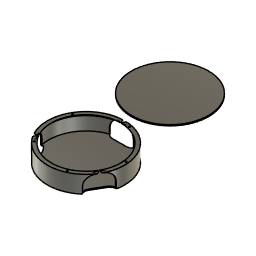
Robotica Volledige Robot3 v2 (Autodesk Fusion 360 design; units mm, degrees)
Autodesk Fusion 360 part; units mm, degrees
sketch "Sketch1" plane through (0, 0, 0) normal (0, 0, 1) x (1, 0, 0)
  circle A0 centre (0, 0) radius 110 construction
  circle A1 centre (0, 0) radius 105.5
  line L0 (-15, 90.5) -> (15, 90.5)
  line L1 (15, 90.5) -> (15, 27.5)
  line L2 (15, 27.5) -> (-15, 27.5)
  line L3 (-15, 27.5) -> (-15, 90.5)
  circle A2 centre (0, 0) radius 102.5
  spline S0 degree 5 poles (-32.987289, 97.046838) (-32.40075, 96.649596) (-31.292492, 95.840182) (-29.823347, 94.581605) (-27.997387, 92.904069) (-24.704967, 91.250774) (-19.527486, 90.398038) (-12.348654, 90.46258) (-5.577784, 90.79374) (-0.094558, 91.003458) (4.346465, 90.964526) (8.472499, 90.723353) (13.019743, 90.460618) (18.177004, 90.44585) (23.049454, 90.978092) (27.290126, 92.192845) (30.008132, 93.760088) (31.651296, 95.273016) (32.571175, 96.430723) (32.987289, 97.046838) knots 0 0 0 0 0 0 0.06666667 0.13333333 0.2 0.26666667 0.33333333 0.4 0.46666667 0.53333333 0.6 0.66666667 0.73333333 0.8 0.86666667 0.93333333 1 1 1 1 1 1
  line L4 (8, 90.5) -> (22, 90.5)
  line L5 (-37.716487, 100.249751) -> (-28.258092, 93.843924)
  line L6 (-24.570837, 90.5) -> (-5.429163, 90.5)
  line L7 (-70.875299, -58.240381) -> (-85.875299, -32.259619)
  line L8 (-16.315699, -26.740381) -> (-70.875299, -58.240381)
  line L9 (-85.875299, -32.259619) -> (-31.315699, -0.759619)
  line L10 (-31.315699, -0.759619) -> (-16.315699, -26.740381)
  spline S1 degree 5 poles (-67.551382, -77.091249) (-67.500631, -76.384671) (-67.353787, -75.020184) (-66.998399, -73.118579) (-66.45859, -70.698483) (-66.673005, -67.020516) (-68.523255, -62.110318) (-72.168565, -55.925538) (-75.840794, -50.227373) (-78.764027, -45.583618) (-80.950823, -41.718114) (-82.804978, -38.024277) (-84.851065, -33.954881) (-87.416906, -29.481178) (-90.314066, -25.527634) (-93.486409, -22.46248) (-96.202684, -20.89224) (-98.3345, -20.225682) (-99.797043, -20.007896) (-100.538672, -19.955588) knots 0 0 0 0 0 0 0.06666667 0.13333333 0.2 0.26666667 0.33333333 0.4 0.46666667 0.53333333 0.6 0.66666667 0.73333333 0.8 0.86666667 0.93333333 1 1 1 1 1 1
  line L11 (85.875299, -32.259619) -> (70.875299, -58.240381)
  line L12 (31.315699, -0.759619) -> (85.875299, -32.259619)
  line L13 (70.875299, -58.240381) -> (16.315699, -26.740381)
  line L14 (16.315699, -26.740381) -> (31.315699, -0.759619)
  spline S2 degree 5 poles (100.538672, -19.955588) (99.901381, -20.264925) (98.646278, -20.819998) (96.821746, -21.463026) (94.455977, -22.205586) (91.377972, -24.230258) (88.050741, -28.28772) (84.517219, -34.537042) (81.418577, -40.566368) (78.858585, -45.419839) (76.604358, -49.246412) (74.332479, -52.699076) (71.831322, -56.505737) (69.239902, -60.964672) (67.264612, -65.450459) (66.196283, -69.730365) (66.194552, -72.867849) (66.683204, -75.047334) (67.225868, -76.422826) (67.551382, -77.091249) knots 0 0 0 0 0 0 0.06666667 0.13333333 0.2 0.26666667 0.33333333 0.4 0.46666667 0.53333333 0.6 0.66666667 0.73333333 0.8 0.86666667 0.93333333 1 1 1 1 1 1
  line L15 (-32.987289, 97.046838) -> (-33.952771, 99.887233)
  line L16 (32.987289, 97.046838) -> (33.952771, 99.887233)
  line L17 (100.538672, -19.955588) -> (103.481267, -20.539654)
  line L18 (67.551382, -77.091249) -> (69.528496, -79.347579)
  line L19 (-67.551382, -77.091249) -> (-69.528496, -79.347579)
  line L20 (-100.538672, -19.955588) -> (-103.481267, -20.539654)
  dimension "d1" = 220
  dimension "d2" = 211
  dimension "d5" = -3
  dimension "d8" = 360
  dimension "d9" = 3
  dimension "d10" = 3
  dimension "d11" = 3
  dimension "d12" = 3
  dimension "d13" = 3
  dimension "d14" = 3
  constraint coincident A0.centre A1.centre
  constraint concentric A0 A1
  constraint horizontal L0
  constraint vertical L1
  constraint horizontal L2
  constraint vertical L3
  constraint midpoint L0.end L4
  constraint coincident L0 L4.start
  constraint midpoint L0.start L6
  measures "d1" diameter of A0
  measures "d2" diameter of A1
extrude "Extrude1" add sketch "Sketch1" against normal blind 3 contours A1 A2 L16 L17 | A1 L5 L15 | L1 L2 L3 A2 S0 L8 L9 L10 S1 L12 L13 L14 S2 | A1 A2 L18 L19 | A1 A2 L5 L20 | L0 L1 L2 L3 L4 L6 | L11 L12 L13 L14 | L7 L8 L9 L10 picked at (93.399703, 46.371336) picked at (-33.867602, 98.859051) picked at (-32.708198, 67.519481) picked at (64.836769, -81.645797) picked at (-38.542877, 95.833138) picked at (-1.809721, 48.5) picked at (62.688766, -30.419873) picked at (-39.502232, -28.580127) makes body 1
extrude "Extrude2" add sketch "Sketch1" along normal blind 44 contours A1 A2 L16 L17 | A1 L5 L15 | A1 A2 L18 L19 | A1 A2 L5 L20 picked at (93.399703, 46.371336) picked at (-33.867602, 98.859051) picked at (64.836769, -81.645797) picked at (-38.542877, 95.833138) bodies 1
sketch "Sketch2" plane through (0, 0, 44) normal (0, 0, 1) x (-1, 0, 0)
  arc A0 (-100.538672, 19.955588) -> (-32.987289, -97.046838) centre (0, 0) ccw
  line L0 (-100.538672, 19.955588) -> (-103.481267, 20.539654)
  arc A1 (-103.481267, 20.539654) -> (-33.952771, -99.887233) centre (0, 0) ccw
  line L1 (-33.952771, -99.887233) -> (-32.987289, -97.046838)
  circle A2 centre (0, 0) radius 105.5
  dimension "d19" = 211
  constraint concentric A0 A2
  measures "d19" diameter of A2
extrude "Extrude3" add sketch "Sketch2" along normal blind 3 contours A0 L0 L1 A2 | A0 L0 A1 L1 A2 picked at (-15.270239, -6.157135) picked at (-78.66347, -68.424421) bodies 1
fillet "Fillet1" radius 7.5 3 edges at (0, -102.5, 44) (-88.767604, 51.25, 44) (88.767604, 51.25, 44) on bodies 1
fillet "Fillet2" radius 30 6 edges at (32.263178, 94.916541, 44) (-32.263178, 94.916541, 44) (66.068547, -75.399003, 44) (98.331725, -19.517539, 44) (-98.331725, -19.517539, 44) (-66.068547, -75.399003, 44) on bodies 1
ref_plane "WorkPlane1" through (0, 0, 44) normal (0, 0, 1) x (-1, 0, 0)
split "Split1" by plane through (0, 0, 44) normal (0, 0, 1) bodies 1 makes body 2 at (23.267657, 16.475731, 47)
move_body "Move1" bodies 2 to x (1, 0, 0) y (0, 1, 0) z (0, 0, 1) at (0, 230, 0)
sketch "Sketch4" plane through (0, 0, 44) normal (0, 0, 1) x (-1, 0, 0)
  arc A0 (89.22148, 56.300778) -> (-89.22148, 56.300778) centre (0, 0) ccw
  line L0 (-89.22148, 56.300778) -> (-81.968164, 48.023121)
  arc A1 (81.968164, 48.023121) -> (-81.968164, 48.023121) centre (0, 0) ccw
  line L1 (81.968164, 48.023121) -> (89.22148, 56.300778)
  line L2 (0, 0) -> (100.25, 0) construction
  circle A2 centre (86.819047, -50.125) radius 2
  circle A3 centre (74.500269, 67.080343) radius 2
  circle A4 centre (-40.775348, 91.582932) radius 2
  circle A5 centre (-99.70082, -10.478978) radius 2
  circle A6 centre (-20.843147, -98.059297) radius 2
  dimension "d38" = 4
  dimension "d40" = 360
  constraint horizontal L2
  measures "d38" diameter of A2
hole "Hole1" at (-86.819047, 50.125, 44) at (-74.500269, -67.080343, 44) at (40.775348, -91.582932, 44) at (99.70082, 10.478978, 44) at (20.843147, 98.059297, 44) direction (0, 0, -1) diameter 4 depth 7 tip angle 180 bodies 1
